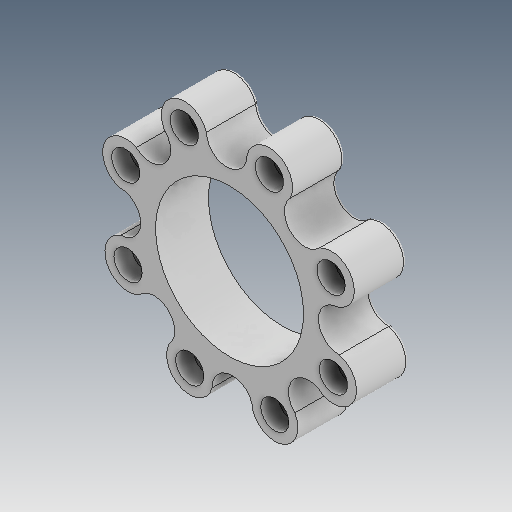
# Autodesk Inventor part: Cycloidal gear 02
Saved by Autodesk Inventor 2020.3 (Build 243373010, 373A)
## iProperties
Created: 2021-05-01
Part Number: Cycloidal gear 02
Material: Generic
Document SubType Name: Modeling
Designer: marti
Density: 1 g/cm^3
Appearance: Default
Author: marti
Autodesk Inventor part; units mm, degrees
ref_plane "YZ Plane" through (0, 0, 0) normal (1, 0, 0) x (0, 1, 0)
ref_plane "XZ Plane" through (0, 0, 0) normal (0, 1, 0) x (-1, 0, 0)
ref_plane "XY Plane" through (0, 0, 0) normal (0, 0, 1) x (1, 0, 0)
sketch "Sketch1" plane through (0, 0, 0) normal (0, 0, 1) x (1, 0, 0)
  circle A0 centre (0, 0) radius 25
  line L0 (0, 0) -> (-11.961, 26.8649)
  line L1 (0, 0) -> (-16.8529, 23.196)
  arc A1 (-6.5977, 30.8649) -> (-18.5223, 25.5557) centre (-12.8375, 28.8334) ccw
  circle A2 centre (0, 0) radius 31.5621
  line L2 (0, 0) -> (0, 31.5621)
  line L3 (0, 0) -> (-5.1978, 24.4537)
  arc A3 (-26.49, 17.1595) -> (-31.1678, 4.9733) centre (-29.4658, 11.3109) ccw
  arc A4 (-30.8649, -6.5977) -> (-25.5557, -18.5223) centre (-28.8334, -12.8375) ccw
  arc A5 (-17.1595, -26.49) -> (-4.9733, -31.1678) centre (-11.3109, -29.4658) ccw
  arc A6 (6.5977, -30.8649) -> (18.5223, -25.5557) centre (12.8375, -28.8334) ccw
  arc A7 (26.49, -17.1595) -> (31.1678, -4.9733) centre (29.4658, -11.3109) ccw
  arc A8 (30.8649, 6.5977) -> (25.5557, 18.5223) centre (28.8334, 12.8375) ccw
  arc A9 (17.1595, 26.49) -> (4.9733, 31.1678) centre (11.3109, 29.4658) ccw
  arc A10 (-6.5977, 30.8649) -> (4.9733, 31.1678) centre (-0.8122, 31.0164) ccw
  arc A11 (-26.49, 17.1595) -> (-18.5223, 25.5557) centre (-22.5062, 21.3576) ccw
  arc A12 (-30.8649, -6.5977) -> (-31.1678, 4.9733) centre (-31.0164, -0.8122) ccw
  arc A13 (-17.1595, -26.49) -> (-25.5557, -18.5223) centre (-21.3576, -22.5062) ccw
  arc A14 (6.5977, -30.8649) -> (-4.9733, -31.1678) centre (0.8122, -31.0164) ccw
  arc A15 (26.49, -17.1595) -> (18.5223, -25.5557) centre (22.5062, -21.3576) ccw
  arc A16 (30.8649, 6.5977) -> (31.1678, -4.9733) centre (31.0164, 0.8122) ccw
  arc A17 (17.1595, 26.49) -> (25.5557, 18.5223) centre (21.3576, 22.5062) ccw
  point P0 (-18.5223, 25.5557)
  point P1 (-26.49, 17.1595)
  point P2 (-31.1678, 4.9733)
  point P3 (-30.8649, -6.5977)
  point P4 (-25.5557, -18.5223)
  point P5 (-17.1595, -26.49)
  point P6 (-4.9733, -31.1678)
  point P7 (6.5977, -30.8649)
  point P8 (18.5223, -25.5557)
  point P9 (26.49, -17.1595)
  point P10 (31.1678, -4.9733)
  point P11 (30.8649, 6.5977)
  point P12 (25.5557, 18.5223)
  point P13 (17.1595, 26.49)
  point P14 (4.9733, 31.1678)
  dimension "d0" = 50
  dimension "d29" = 12
  dimension "d36" = 24
  dimension "d41" = 360
  dimension "d45" = 360
  constraints: 37 point on circle, 17 centre point, 8 end point, 3 coincident, 1 point on line, 1 tangent, 1 vertical, 70 other
  measures "d29" angle of L1 L0
  measures "d36" angle of L3 L1
extrude "Extrusion3" add sketch "Sketch1" along normal mid plane 15 contours A0 L1 L2 | L2 L3 A0 | A0 L0 L1 | L3 L0 A0
extrude "Extrusion4" add sketch "Sketch1" along normal mid plane 15 contours A10 A2 A17 A16 A15 A14 A13 A12 A11 | A2 A1 | A9 A2 | A2 A3 | A8 A2 | A2 A4 | A7 A2 | A2 A5 | A6 A2
fillet "Fillet2" radius 1 16 edges at (-35.5921, 13.6625, -7.5) (-18.3081, 17.3737, -7.5) (-15.5065, 34.8283, -7.5) (-0.6607, 25.2309, -7.5) (13.6625, 35.5921, -7.5) (17.3737, 18.3081, -7.5) (34.8283, 15.5065, -7.5) (25.2309, 0.6607, -7.5) (35.5921, -13.6625, -7.5) (18.3081, -17.3737, -7.5) (15.5065, -34.8283, -7.5) (0.6607, -25.2309, -7.5) (-13.6625, -35.5921, -7.5) (-17.3737, -18.3081, -7.5) (-34.8283, -15.5065, -7.5) (-25.2309, -0.6607, -7.5)
sketch "Sketch3" plane through (0, 0, -7.5) normal (0, 0, -1) x (-1, 0, 0)
  circle A0 centre (0, 0) radius 21
  dimension "d50" = 42
  constraints: 1 centre point, 1 coincident
  measures "d50" diameter of A0
extrude "Extrusion5" cut sketch "Sketch3" against normal through all
sketch "Sketch4" plane through (0, 0, 7.5) normal (0, 0, 1) x (1, 0, 0)
  arc A0 (-6.5977, 30.8649) -> (-18.5223, 25.5557) centre (-12.8375, 28.8334) ccw projected
  arc A1 (-6.5977, 30.8649) -> (4.9733, 31.1678) centre (-0.8122, 31.0164) ccw projected
  arc A2 (17.1595, 26.49) -> (4.9733, 31.1678) centre (11.3109, 29.4658) ccw projected
  arc A3 (17.1595, 26.49) -> (25.5557, 18.5223) centre (21.3576, 22.5062) ccw projected
  arc A4 (30.8649, 6.5977) -> (25.5557, 18.5223) centre (28.8334, 12.8375) ccw projected
  arc A5 (30.8649, 6.5977) -> (31.1678, -4.9733) centre (31.0164, 0.8122) ccw projected
  arc A6 (26.49, -17.1595) -> (31.1678, -4.9733) centre (29.4658, -11.3109) ccw projected
  arc A7 (26.49, -17.1595) -> (18.5223, -25.5557) centre (22.5062, -21.3576) ccw projected
  arc A8 (6.5977, -30.8649) -> (18.5223, -25.5557) centre (12.8375, -28.8334) ccw projected
  arc A9 (6.5977, -30.8649) -> (-4.9733, -31.1678) centre (0.8122, -31.0164) ccw projected
  arc A10 (-17.1595, -26.49) -> (-4.9733, -31.1678) centre (-11.3109, -29.4658) ccw projected
  arc A11 (-17.1595, -26.49) -> (-25.5557, -18.5223) centre (-21.3576, -22.5062) ccw projected
  arc A12 (-30.6817, -7.5914) -> (-26.1716, -17.7213) centre (-28.8334, -12.8375) ccw projected
  arc A13 (-30.8649, -6.5977) -> (-25.5557, -18.5223) centre (-28.8334, -12.8375) ccw projected
  arc A14 (-30.8649, -6.5977) -> (-31.1678, 4.9733) centre (-31.0164, -0.8122) ccw projected
  arc A15 (-26.49, 17.1595) -> (-31.1678, 4.9733) centre (-29.4658, 11.3109) ccw projected
  arc A16 (-26.49, 17.1595) -> (-18.5223, 25.5557) centre (-22.5062, 21.3576) ccw projected
  point P0 (0, 0)
sketch "Sketch8" plane through (0, 0, 7.5) normal (0, 0, 1) x (1, 0, 0)
  circle A0 centre (0, 0) radius 21 projected
  arc A1 (-26.49, 17.1595) -> (-31.1678, 4.9733) centre (-29.4658, 11.3109) ccw projected
  arc A2 (-30.8649, -6.5977) -> (-31.1678, 4.9733) centre (-31.0164, -0.8122) ccw projected
  arc A3 (-30.8649, -6.5977) -> (-25.5557, -18.5223) centre (-28.8334, -12.8375) ccw projected
  arc A4 (-17.1595, -26.49) -> (-25.5557, -18.5223) centre (-21.3576, -22.5062) ccw projected
  arc A5 (-17.1595, -26.49) -> (-4.9733, -31.1678) centre (-11.3109, -29.4658) ccw projected
  arc A6 (6.5977, -30.8649) -> (-4.9733, -31.1678) centre (0.8122, -31.0164) ccw projected
  arc A7 (6.5977, -30.8649) -> (18.5223, -25.5557) centre (12.8375, -28.8334) ccw projected
  arc A8 (26.49, -17.1595) -> (18.5223, -25.5557) centre (22.5062, -21.3576) ccw projected
  arc A9 (26.49, -17.1595) -> (31.1678, -4.9733) centre (29.4658, -11.3109) ccw projected
  arc A10 (30.8649, 6.5977) -> (31.1678, -4.9733) centre (31.0164, 0.8122) ccw projected
  arc A11 (30.8649, 6.5977) -> (25.5557, 18.5223) centre (28.8334, 12.8375) ccw projected
  arc A12 (17.1595, 26.49) -> (25.5557, 18.5223) centre (21.3576, 22.5062) ccw projected
  arc A13 (17.1595, 26.49) -> (4.9733, 31.1678) centre (11.3109, 29.4658) ccw projected
  arc A14 (-6.5977, 30.8649) -> (4.9733, 31.1678) centre (-0.8122, 31.0164) ccw projected
  arc A15 (-6.5977, 30.8649) -> (-18.5223, 25.5557) centre (-12.8375, 28.8334) ccw projected
  arc A16 (-26.49, 17.1595) -> (-18.5223, 25.5557) centre (-22.5062, 21.3576) ccw projected
  constraints: 1 coincident
hole "Hole1" at (-12.8375, 28.8334, 7.5) direction (0, 0, -1) diameter 5 end through all counterbore diameter 8 counterbore depth 5
pattern_circular "Circular Pattern2" count 8 over 360 about axis through (0, 0, -10) along (0, 0, 1) of "Hole1"
sketch "Sketch9" plane through (0, 0, 7.5) normal (0, 0, 1) x (1, 0, 0)
  circle A0 centre (-12.8375, 28.8334) radius 2.5 projected
  circle A1 centre (11.3109, 29.4658) radius 2.5 projected
  circle A2 centre (28.8334, 12.8375) radius 2.5 projected
  circle A3 centre (29.4658, -11.3109) radius 2.5 projected
  circle A4 centre (12.8375, -28.8334) radius 2.5 projected
  circle A5 centre (-11.3109, -29.4658) radius 2.5 projected
  circle A6 centre (-28.8334, -12.8375) radius 2.5 projected
  circle A7 centre (-29.4658, 11.3109) radius 2.5 projected
  point P0 (0, 0)
body "Solid2"
